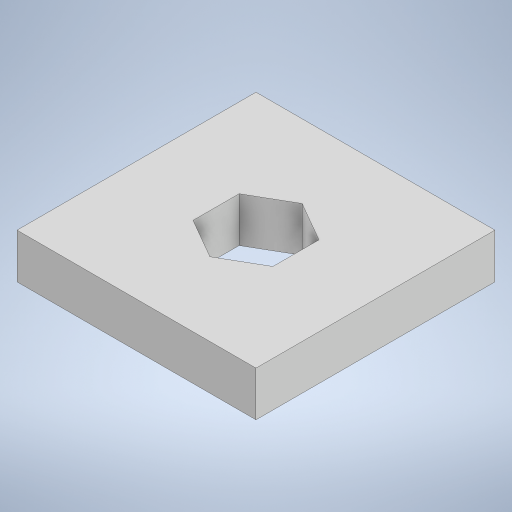
# Autodesk Inventor part: Hex Box +2mm
Saved by Autodesk Inventor 2023 (Build 270158000, 158)
## iProperties
Created: 2023-01-21
Part Number: Hex Box +2mm
Material: Generic
Document SubType Name: Modeling
Designer: bugme
Density: 1 g/cm^3
Appearance: Default
Author: bugme
Autodesk Inventor part; units mm, degrees
ref_plane "YZ Plane" through (0, 0, 0) normal (1, 0, 0) x (0, 1, 0)
ref_plane "XZ Plane" through (0, 0, 0) normal (0, 1, 0) x (-1, 0, 0)
ref_plane "XY Plane" through (0, 0, 0) normal (0, 0, 1) x (1, 0, 0)
sketch "Sketch1" plane through (0, 0, 0) normal (0, 1, 0) x (-1, 0, 0)
  line L0 (7.9861, 7.7649) -> (7.9861, -43.0351)
  line L1 (7.9861, -43.0351) -> (-42.8139, -43.0351)
  line L2 (-42.8139, -43.0351) -> (-42.8139, 7.7649)
  line L3 (-42.8139, 7.7649) -> (7.9861, 7.7649)
  line L4 (-17.4139, -27.4351) -> (-25.901, -22.5351)
  line L5 (-25.901, -22.5351) -> (-25.901, -12.7351)
  line L6 (-25.901, -12.7351) -> (-17.4139, -7.8351)
  line L7 (-17.4139, -7.8351) -> (-8.9269, -12.7351)
  line L8 (-8.9269, -12.7351) -> (-8.9269, -22.5351)
  line L9 (-8.9269, -22.5351) -> (-17.4139, -27.4351)
  point P0 (0, 0)
  point P1 (-17.4139, -17.6351)
  point P2 (-21.6575, -24.9851)
  point P3 (-13.1704, -10.2851)
  dimension "d0" = 50.8
  dimension "d1" = 50.8
  dimension "d2" = 14.7
  constraints: 20 end point, 3 perpendicular, 2 midpoint, 1 vertical, 13 other
  measures "d0" distance of L0.start L0.end
  measures "d1" distance of L0.end L1.end
  measures "d2" vertical distance of point (-21.657, -24.985) point (-13.17, -10.285)
extrude "Extrusion1" add sketch "Sketch1" along normal blind 9.525
body "Solid1"
